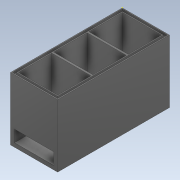
# Autodesk Inventor part: EierkocherTeil1
Saved by Autodesk Inventor 2020 (Build 240168000, 168)
## iProperties
Created: 2022-01-25
Part Number: EierkocherTeil1
Material: Acetalharz, Schwarz
Document SubType Name: Modeling
Designer: Julian Uhl
Density: 1.425 g/cm^3
Appearance: Glatt - Schwarz
Author: Julian Uhl
Autodesk Inventor part; units mm, degrees
ref_plane "YZ Plane" through (0, 0, 0) normal (1, 0, 0) x (0, 1, 0)
ref_plane "XZ Plane" through (0, 0, 0) normal (0, 1, 0) x (-1, 0, 0)
ref_plane "XY Plane" through (0, 0, 0) normal (0, 0, 1) x (1, 0, 0)
sketch "Skizze1" plane through (0, 0, 0) normal (0, 0, 1) x (1, 0, 0)
  line L0 (-24, 0) -> (144, 0) projected
  line L1 (0, -32) -> (0, 192) projected
  line L2 (0, 0) -> (120, 0)
  line L3 (120, 0) -> (120, 160)
  line L4 (120, 160) -> (0, 160)
  line L5 (0, 160) -> (0, 0)
  point P0 (0, 160)
  dimension "d0" = 120
  dimension "d1" = 160
  constraints: 8 end point, 2 parallel, 1 horizontal, 1 perpendicular
  measures "d0" distance between parallel lines of L3 L1
  measures "d1" distance between parallel lines of L2 L4
extrude "Extrusion1" add sketch "Skizze1" along normal blind 285
sketch "Skizze2" plane through (0, 160, 0) normal (0, 1, 0) x (1, 0, 0)
  point P0 (0, 0)
sketch "Skizze3" plane through (0, 0, 285) normal (0, 0, 1) x (1, 0, 0)
  line L0 (10, 40) -> (110, 40)
  line L1 (110, 40) -> (110, 10)
  line L2 (110, 10) -> (10, 10)
  line L3 (10, 10) -> (10, 40)
  line L4 (0, 0) -> (120, 0) projected
  line L5 (120, 0) -> (120, 160) projected
  line L6 (0, 160) -> (0, 0) projected
  dimension "d4" = 10
  dimension "d5" = 10
  dimension "d6" = 10
  dimension "d7" = 30
  constraints: 8 end point, 2 parallel, 1 horizontal, 1 perpendicular
  measures "d4" distance between parallel lines of L4 L2
  measures "d5" distance between parallel lines of L5 L1
  measures "d6" distance between parallel lines of L6 L3
  measures "d7" distance between parallel lines of L2 L0
extrude "Extrusion2" cut sketch "Skizze3" against normal blind 275
sketch "Skizze4" plane through (0, 160, 0) normal (0, 1, 0) x (1, 0, 0)
  point P0 (0, 0)
sketch "Skizze5" plane through (0, 160, 0) normal (0, 1, 0) x (1, 0, 0)
  line L0 (10, -10) -> (110, -10)
  line L1 (110, -10) -> (110, -275)
  line L2 (110, -275) -> (10, -275)
  line L3 (10, -275) -> (10, -10)
  line L4 (10, -190) -> (110, -190)
  line L5 (120, 0) -> (0, 0) projected
  line L6 (10, -100) -> (110, -100)
  line L7 (10, -185) -> (110, -185)
  line L8 (120, -285) -> (0, -285) projected
  line L9 (10, -95) -> (110, -95)
  line L10 (0, 0) -> (0, -285) projected
  line L11 (120, 0) -> (120, -285) projected
  dimension "d10" = 10
  dimension "d11" = 10
  dimension "d12" = 5
  dimension "d13" = 85
  dimension "d14" = 85
  dimension "d15" = 5
  dimension "d16" = 85
  dimension "d17" = 10
  dimension "d18" = 10
  constraints: 16 end point, 8 point on line, 5 perpendicular, 2 parallel, 1 horizontal
  measures "d10" distance between parallel lines of L0 L5
  measures "d11" distance between parallel lines of L2 L8
  measures "d12" distance between parallel lines of L7 L4
  measures "d13" distance between parallel lines of L2 L4
  measures "d14" distance between parallel lines of L7 L6
  measures "d15" distance between parallel lines of L6 L9
  measures "d16" distance between parallel lines of L9 L0
  measures "d17" distance between parallel lines of L10 L3
  measures "d18" distance between parallel lines of L11 L1
extrude "Extrusion3" cut sketch "Skizze5" against normal blind 110 contours L0 L1 L9 L3 | L6 L1 L7 L3 | L4 L1 L2 L3
sketch "Skizze6" plane through (0, 160, 0) normal (0, 1, 0) x (1, 0, 0)
  line L0 (7.5, -7.5) -> (112.5, -7.5)
  line L1 (112.5, -7.5) -> (112.5, -277.5)
  line L2 (112.5, -277.5) -> (7.5, -277.5)
  line L3 (7.5, -277.5) -> (7.5, -7.5)
  line L4 (2.5, -2.5) -> (117.5, -2.5)
  line L5 (117.5, -2.5) -> (117.5, -282.5)
  line L6 (117.5, -282.5) -> (2.5, -282.5)
  line L7 (2.5, -282.5) -> (2.5, -2.5)
  line L8 (120, 0) -> (120, -285) projected
  line L9 (110, -190) -> (110, -275) projected
  line L10 (110, -275) -> (10, -275) projected
  line L11 (120, -285) -> (0, -285) projected
  line L12 (10, -275) -> (10, -190) projected
  line L13 (0, 0) -> (0, -285) projected
  line L14 (120, 0) -> (0, 0) projected
  line L15 (10, -10) -> (110, -10) projected
  dimension "d21" = 2.5
  dimension "d22" = 2.5
  dimension "d23" = 2.5
  dimension "d24" = 2.5
  dimension "d25" = 2.5
  dimension "d26" = 2.5
  dimension "d27" = 2.5
  dimension "d28" = 2.5
  constraints: 16 end point, 4 parallel, 2 horizontal, 2 perpendicular
  measures "d21" distance between parallel lines of L8 L5
  measures "d22" distance between parallel lines of L1 L9
  measures "d23" distance between parallel lines of L10 L2
  measures "d24" distance between parallel lines of L11 L6
  measures "d25" distance between parallel lines of L12 L3
  measures "d26" distance between parallel lines of L7 L13
  measures "d27" distance between parallel lines of L14 L4
  measures "d28" distance between parallel lines of L15 L0
extrude "Extrusion4" cut sketch "Skizze6" against normal blind 5 contours L4 L5 L6 L7
